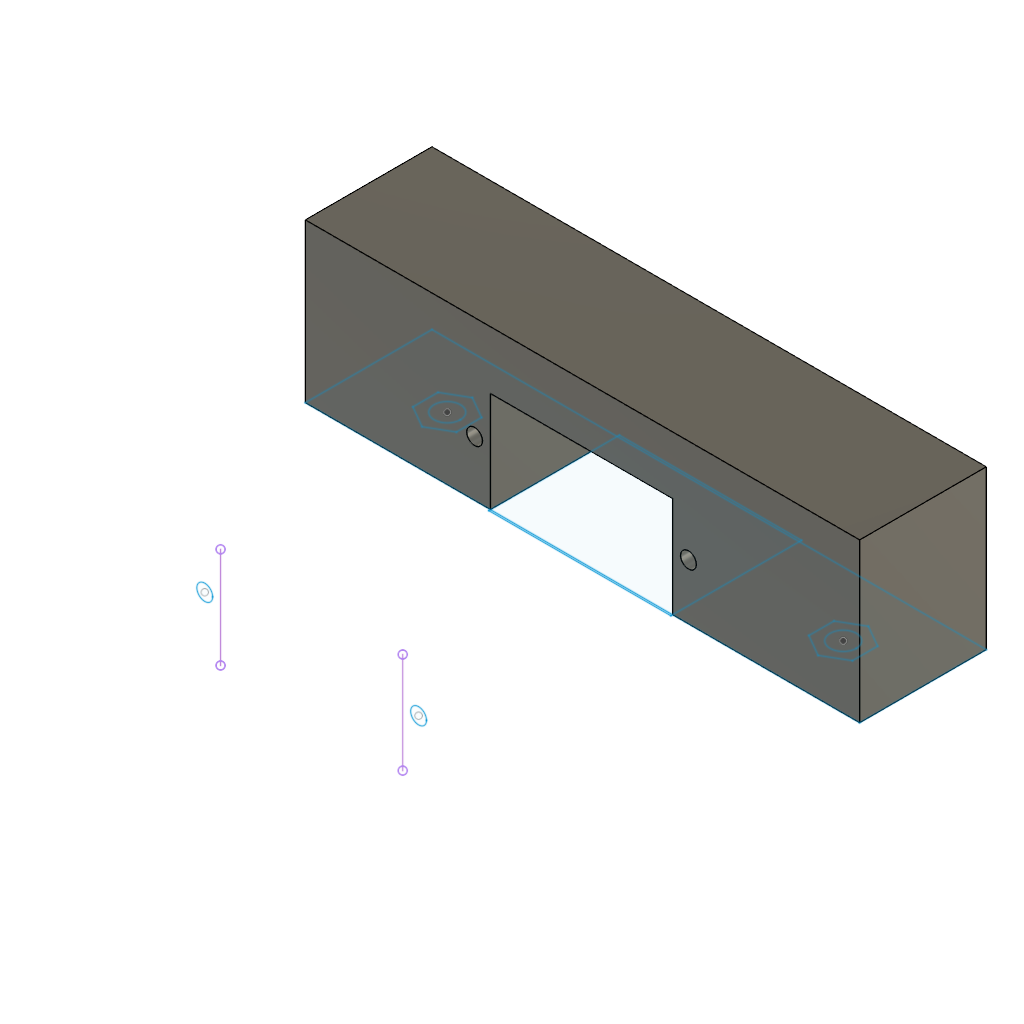
seminaire_FISA-A3_fixation_servomoteur (Autodesk Fusion 360 design; units mm, degrees)
part number: 2026-09-07-13-34-24-019
Autodesk Fusion 360 part; units mm, degrees
sketch "Esquisse1" plane through (0, 0, 0) normal (0, 0, 1) x (1, 0, 0)
  line L0 (-50, 50.0735) -> (20, 50.0735)
  line L1 (20, 50.0735) -> (20, 34.0735)
  line L2 (20, 34.0735) -> (-50, 34.0735)
  line L3 (-50, 34.0735) -> (-50, 50.0735)
  circle A0 centre (-40, 42) radius 1.65
  circle A1 centre (10, 42) radius 1.65
  line L4 (7.25, 40.4123) -> (10, 38.8246)
  line L5 (10, 38.8246) -> (12.75, 40.4123)
  line L6 (12.75, 40.4123) -> (12.75, 43.5877)
  line L7 (12.75, 43.5877) -> (10, 45.1754)
  line L8 (10, 45.1754) -> (7.25, 43.5877)
  line L9 (7.25, 43.5877) -> (7.25, 40.4123)
  line L10 (-42.75, 40.4123) -> (-40, 38.8246)
  line L11 (-40, 38.8246) -> (-37.25, 40.4123)
  line L12 (-37.25, 40.4123) -> (-37.25, 43.5877)
  line L13 (-37.25, 43.5877) -> (-40, 45.1754)
  line L14 (-40, 45.1754) -> (-42.75, 43.5877)
  line L15 (-42.75, 43.5877) -> (-42.75, 40.4123)
  point P0 (10, 42)
  point P1 (-40, 42)
  dimension "d2" = 16
  dimension "d3" = 70
  dimension "d5" = 3.3
  dimension "d6" = 3.3
  dimension "d7" = 10
  dimension "d8" = 10
  dimension "d23" = 2.75
  dimension "d24" = 2.75
  dimension "d37" = 50
  constraint horizontal L0
  constraint vertical L1
  constraint horizontal L2
  constraint vertical L3
  constraint coincident P0 A1.centre
  constraint coincident P1 A0.centre
  measures "d2" distance of L0.end L1.end
  measures "d3" distance of L1.end L2.end
  measures "d5" diameter of A0
  measures "d6" diameter of A1
  measures "d7" distance of L3 P1
  measures "d8" distance of L1 P0
  measures "d23" distance of P0 L9
  measures "d24" distance of P1 L15
  measures "d37" distance of P0 P1
extrude "Extrusion1" add sketch "Esquisse1" along normal blind 20 contours L0 L1 L2 L3 | A0 | A1 | L4 L5 L6 L7 L8 L9 | L10 L11 L12 L13 L14 L15
extrude "Extrusion7" cut sketch "Esquisse1" along normal blind 19 and the other way blind 0 contours A0 | A1
extrude "Extrusion6" cut sketch "Esquisse1" along normal blind 13 and the other way blind -11 contours L4 L5 L6 L7 L8 L9 | L10 L11 L12 L13 L14 L15
sketch "Esquisse2" plane through (0, 0, 0) normal (0, 0, 1) x (1, 0, 0)
  line L0 (-26.6171, 50.3546) -> (-3.6171, 50.3546)
  line L1 (-3.6171, 50.3546) -> (-3.6171, 33.8546)
  line L2 (-3.6171, 33.8546) -> (-26.6171, 33.8546)
  line L3 (-26.6171, 33.8546) -> (-26.6171, 50.3546)
  dimension "d11" = 23
  dimension "d12" = 16.5
  constraint horizontal L0
  constraint vertical L1
  constraint horizontal L2
  constraint vertical L3
  measures "d11" distance of L1.end L2.end
  measures "d12" distance of L0 L2
extrude "Extrusion2" cut sketch "Esquisse2" along normal blind 12.7
sketch "Esquisse3" plane through (0, 0, 0) normal (0, 1, 0) x (1, 0, 0)
  circle A0 centre (-28.6171, -7) radius 1
  circle A1 centre (-1.6171, -7) radius 1
  line L0 (-26.6171, 0) -> (-26.6171, -12.7)
  line L1 (-3.6171, -12.7) -> (-3.6171, 0)
  dimension "d15" = 2
  dimension "d16" = 2
  dimension "d17" = 2
  dimension "d18" = 2
  measures "d15" diameter of A0
  measures "d16" diameter of A1
  measures "d17" distance of A0.centre L0
  measures "d18" distance of A1.centre L1
extrude "Extrusion3" cut sketch "Esquisse3" along normal blind 51 and the other way blind -34
extrude "Extrusion4" cut sketch "Esquisse1" along normal blind 8 and the other way blind -5 contours L10 L11 L12 L13 L14 L15
extrude "Extrusion5" cut sketch "Esquisse1" along normal blind 8 and the other way blind -5 contours L4 L5 L6 L7 L8 L9
equation "d6 = d5"
equation "d16 = d15"
